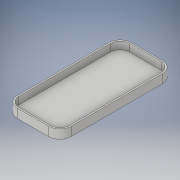
# Autodesk Inventor part: HandyHuelleMitText
Saved by Autodesk Inventor 2018 (Build 220112000, 112)
## iProperties
Created: 2017-06-18
Part Number: HandyHuelleMitText
Material: Generisch
Document SubType Name: Modeling
Designer: Ich
Density: 1 g/cm^3
Appearance: Vorgabe
Author: Ich
Autodesk Inventor part; units mm, degrees
ref_plane "YZ Plane" through (0, 0, 0) normal (1, 0, 0) x (0, 1, 0)
ref_plane "XZ Plane" through (0, 0, 0) normal (0, 1, 0) x (-1, 0, 0)
ref_plane "XY Plane" through (0, 0, 0) normal (0, 0, 1) x (1, 0, 0)
sketch "Skizze1" plane through (0, 0, 0) normal (0, 0, 1) x (1, 0, 0)
  line L0 (21, -76.5) -> (-21, -76.5)
  line L1 (-36, -61.5) -> (-36, 61.5)
  line L2 (-21, 76.5) -> (21, 76.5)
  line L3 (36, 61.5) -> (36, -61.5)
  line L4 (36, -76.5) -> (-36, 76.5) construction
  line L5 (-36, -76.5) -> (36, 76.5) construction
  arc A0 (-21, 76.5) -> (-36, 61.5) centre (-21, 61.5) ccw
  arc A1 (36, 61.5) -> (21, 76.5) centre (21, 61.5) ccw
  arc A2 (21, -76.5) -> (36, -61.5) centre (21, -61.5) ccw
  arc A3 (-36, -61.5) -> (-21, -76.5) centre (-21, -61.5) ccw
  point P0 (0, 0)
  dimension "d0" = 72
  dimension "d1" = 153
  dimension "d4" = 15
  dimension "d5" = 15
  constraints: 12 end point, 8 point on circle, 8 point on line, 8 tangent, 4 centre point, 2 equal radius, 2 midpoint, 2 parallel, 1 horizontal, 1 perpendicular
  measures "d0" distance between parallel lines of L3 L1
  measures "d1" distance between parallel lines of L0 L2
  measures "d4" radius of A0
  measures "d5" radius of A1
extrude "Extrusion1" add sketch "Skizze1" along normal blind 12
sketch "Skizze2" plane through (0, 0, 12) normal (0, 0, 1) x (1, 0, 0)
  line L0 (21, -74.5) -> (-21, -74.5)
  line L1 (-34, -61.5) -> (-34, 61.5)
  line L2 (-21, 74.5) -> (21, 74.5)
  line L3 (34, 61.5) -> (34, -61.5)
  line L4 (34, -74.5) -> (-34, 74.5) construction
  line L5 (-34, -74.5) -> (34, 74.5) construction
  arc A0 (34, 61.5) -> (21, 74.5) centre (21, 61.5) ccw
  arc A1 (-21, 74.5) -> (-34, 61.5) centre (-21, 61.5) ccw
  arc A2 (-34, -61.5) -> (-21, -74.5) centre (-21, -61.5) ccw
  arc A3 (21, -74.5) -> (34, -61.5) centre (21, -61.5) ccw
  point P0 (0, 0)
  dimension "d6" = 149
  dimension "d7" = 68
  dimension "d8" = 13
  constraints: 12 end point, 8 point on circle, 8 point on line, 8 tangent, 4 centre point, 3 equal radius, 2 midpoint, 2 parallel, 1 horizontal, 1 perpendicular
  measures "d6" distance between parallel lines of L0 L2
  measures "d7" distance between parallel lines of L1 L3
  measures "d8" radius of A0
extrude "Extrusion2" cut sketch "Skizze2" against normal blind 10
sketch "TextSkizze" plane through (0, 0, 0) normal (0, 0, -1) x (-1, 0, 0)
  line L0 (-11.4354, 0) -> (11.4354, 0) construction
  line L1 (11.4354, 0) -> (11.4354, -5.5416) construction
  line L2 (11.4354, -5.5416) -> (-11.4354, -5.5416) construction
  line L3 (-11.4354, -5.5416) -> (-11.4354, 0) construction
  line L4 (0, 88.5147) -> (0, -102.809) construction
  line L5 (-76.4782, 0) -> (138.3762, 0) construction
  line L6 (21, 76.5) -> (-21, 76.5) construction
  arc A0 (-21, 76.5) -> (-36, 61.5) centre (-21, 61.5) ccw construction
  line L7 (-36, 61.5) -> (-36, -61.5) construction
  arc A1 (-36, -61.5) -> (-21, -76.5) centre (-21, -61.5) ccw construction
  line L8 (-21, -76.5) -> (21, -76.5) construction
  arc A2 (21, -76.5) -> (36, -61.5) centre (21, -61.5) ccw construction
  line L9 (36, -61.5) -> (36, 61.5) construction
  arc A3 (36, 61.5) -> (21, 76.5) centre (21, 61.5) ccw construction
  line L10 (-10.2641, -3.5) -> (-10.2641, -0.4141)
  line L11 (-10.2641, -0.4141) -> (-11.4383, -0.4141)
  line L12 (-11.4383, -0.4141) -> (-11.4383, 0)
  line L13 (-11.4383, 0) -> (-8.6247, 0)
  line L14 (-8.6247, 0) -> (-8.6247, -0.4141)
  line L15 (-8.6247, -0.4141) -> (-9.7989, -0.4141)
  line L16 (-9.7989, -0.4141) -> (-9.7989, -3.5)
  line L17 (-9.7989, -3.5) -> (-10.2641, -3.5)
  spline S0 degree 2 poles (-7.164, -3.5596) (-7.7936, -3.5596) (-8.4857, -2.8533) (-8.4857, -2.201) knots 0 0 0 1 2 2 2
  spline S1 degree 2 poles (-8.4857, -2.201) (-8.4857, -1.56) (-7.8135, -0.7998) (-7.2717, -0.7998) knots 0 0 0 1 2 2 2
  spline S2 degree 2 poles (-7.2717, -0.7998) (-7.0278, -0.7998) (-6.6506, -0.9417) (-6.5116, -1.092) knots 0 0 0 1 2 2 2
  spline S3 degree 2 poles (-6.5116, -1.092) (-6.3698, -1.2423) (-6.2195, -1.6763) (-6.2195, -1.9911) knots 0 0 0 1 2 2 2
  line L18 (-6.2195, -1.9911) -> (-6.2195, -2.2322)
  line L19 (-6.2195, -2.2322) -> (-8.0376, -2.2322)
  spline S4 degree 2 poles (-8.0376, -2.2322) (-8.0376, -2.6888) (-7.5781, -3.1738) (-7.1696, -3.1738) knots 0 0 0 1 2 2 2
  spline S5 degree 2 poles (-7.1696, -3.1738) (-7.025, -3.1738) (-6.7442, -3.1086) (-6.6307, -3.0575) knots 0 0 0 1 2 2 2
  spline S6 degree 2 poles (-6.6307, -3.0575) (-6.5116, -3.0008) (-6.3471, -2.9015) (-6.2932, -2.8562) knots 0 0 0 1 2 2 2
  line L20 (-6.2932, -2.8562) -> (-6.2677, -2.8562)
  line L21 (-6.2677, -2.8562) -> (-6.2677, -3.3383)
  spline S7 degree 2 poles (-6.2677, -3.3383) (-6.3443, -3.3695) (-6.5769, -3.4603) (-6.6676, -3.4858) knots 0 0 0 1 2 2 2
  spline S8 degree 2 poles (-6.6676, -3.4858) (-6.7953, -3.5227) (-7.0051, -3.5596) (-7.164, -3.5596) knots 0 0 0 1 2 2 2
  spline S9 degree 2 poles (-6.6506, -1.8947) (-6.6563, -1.716) (-6.73, -1.455) (-6.8009, -1.3671) knots 0 0 0 1 2 2 2
  spline S10 degree 2 poles (-6.8009, -1.3671) (-6.8775, -1.2678) (-7.1186, -1.1629) (-7.2973, -1.1629) knots 0 0 0 1 2 2 2
  spline S11 degree 2 poles (-7.2973, -1.1629) (-7.4731, -1.1629) (-7.7199, -1.2678) (-7.822, -1.3699) knots 0 0 0 1 2 2 2
  spline S12 degree 2 poles (-7.822, -1.3699) (-7.9213, -1.4749) (-8.0234, -1.7273) (-8.0376, -1.8947) knots 0 0 0 1 2 2 2
  line L22 (-8.0376, -1.8947) -> (-6.6506, -1.8947)
  spline S13 degree 2 poles (-5.0623, -3.5624) (-5.326, -3.5624) (-5.7827, -3.4206) (-5.933, -3.3412) knots 0 0 0 1 2 2 2
  line L23 (-5.933, -3.3412) -> (-5.933, -2.8448)
  line L24 (-5.933, -2.8448) -> (-5.9103, -2.8448)
  spline S14 degree 2 poles (-5.9103, -2.8448) (-5.8536, -2.8902) (-5.7004, -2.998) (-5.5728, -3.0575) knots 0 0 0 1 2 2 2
  spline S15 degree 2 poles (-5.5728, -3.0575) (-5.4622, -3.1114) (-5.1899, -3.1908) (-5.0453, -3.1908) knots 0 0 0 1 2 2 2
  spline S16 degree 2 poles (-5.0453, -3.1908) (-4.9403, -3.1908) (-4.6992, -3.1426) (-4.6425, -3.1029) knots 0 0 0 1 2 2 2
  spline S17 degree 2 poles (-4.6425, -3.1029) (-4.5602, -3.049) (-4.4865, -2.9271) (-4.4865, -2.8023) knots 0 0 0 1 2 2 2
  spline S18 degree 2 poles (-4.4865, -2.8023) (-4.4865, -2.6463) (-4.6567, -2.4846) (-4.8751, -2.4307) knots 0 0 0 1 2 2 2
  spline S19 degree 2 poles (-4.8751, -2.4307) (-4.9602, -2.4109) (-5.2324, -2.3541) (-5.3487, -2.3229) knots 0 0 0 1 2 2 2
  spline S20 degree 2 poles (-5.3487, -2.3229) (-5.6494, -2.235) (-5.9217, -1.872) (-5.9217, -1.6139) knots 0 0 0 1 2 2 2
  spline S21 degree 2 poles (-5.9217, -1.6139) (-5.9217, -1.2565) (-5.3856, -0.8112) (-4.9431, -0.8112) knots 0 0 0 1 2 2 2
  spline S22 degree 2 poles (-4.9431, -0.8112) (-4.7247, -0.8112) (-4.2823, -0.919) (-4.132, -1.0012) knots 0 0 0 1 2 2 2
  line L25 (-4.132, -1.0012) -> (-4.132, -1.4749)
  line L26 (-4.132, -1.4749) -> (-4.1547, -1.4749)
  spline S23 degree 2 poles (-4.1547, -1.4749) (-4.3248, -1.3387) (-4.7389, -1.1827) (-4.9517, -1.1827) knots 0 0 0 1 2 2 2
  spline S24 degree 2 poles (-4.9517, -1.1827) (-5.17, -1.1827) (-5.4707, -1.3671) (-5.4707, -1.5515) knots 0 0 0 1 2 2 2
  spline S25 degree 2 poles (-5.4707, -1.5515) (-5.4707, -1.7188) (-5.292, -1.8805) (-5.0935, -1.9315) knots 0 0 0 1 2 2 2
  spline S26 degree 2 poles (-5.0935, -1.9315) (-4.997, -1.9571) (-4.7531, -2.0081) (-4.6198, -2.0393) knots 0 0 0 1 2 2 2
  spline S27 degree 2 poles (-4.6198, -2.0393) (-4.3305, -2.113) (-4.0355, -2.4506) (-4.0355, -2.7427) knots 0 0 0 1 2 2 2
  spline S28 degree 2 poles (-4.0355, -2.7427) (-4.0355, -2.9129) (-4.1688, -3.2135) (-4.2993, -3.3241) knots 0 0 0 1 2 2 2
  spline S29 degree 2 poles (-4.2993, -3.3241) (-4.4383, -3.4404) (-4.7928, -3.5624) (-5.0623, -3.5624) knots 0 0 0 1 2 2 2
  spline S30 degree 2 poles (-2.8301, -3.5511) (-3.1903, -3.5511) (-3.5959, -3.1398) (-3.5959, -2.6945) knots 0 0 0 1 2 2 2
  line L27 (-3.5959, -2.6945) -> (-3.5959, -1.2395)
  line L28 (-3.5959, -1.2395) -> (-3.8937, -1.2395)
  line L29 (-3.8937, -1.2395) -> (-3.8937, -0.8736)
  line L30 (-3.8937, -0.8736) -> (-3.5959, -0.8736)
  line L31 (-3.5959, -0.8736) -> (-3.5959, -0.1191)
  line L32 (-3.5959, -0.1191) -> (-3.1534, -0.1191)
  line L33 (-3.1534, -0.1191) -> (-3.1534, -0.8736)
  line L34 (-3.1534, -0.8736) -> (-2.3394, -0.8736)
  line L35 (-2.3394, -0.8736) -> (-2.3394, -1.2395)
  line L36 (-2.3394, -1.2395) -> (-3.1534, -1.2395)
  line L37 (-3.1534, -1.2395) -> (-3.1534, -2.4903)
  spline S31 degree 2 poles (-3.1534, -2.4903) (-3.1534, -2.6888) (-3.1393, -2.9072) (-3.091, -3.0008) knots 0 0 0 1 2 2 2
  spline S32 degree 2 poles (-3.091, -3.0008) (-3.0513, -3.0831) (-2.8726, -3.1653) (-2.7195, -3.1653) knots 0 0 0 1 2 2 2
  spline S33 degree 2 poles (-2.7195, -3.1653) (-2.6117, -3.1653) (-2.4103, -3.1001) (-2.3649, -3.0802) knots 0 0 0 1 2 2 2
  line L38 (-2.3649, -3.0802) -> (-2.3394, -3.0802)
  line L39 (-2.3394, -3.0802) -> (-2.3394, -3.4773)
  spline S34 degree 2 poles (-2.3394, -3.4773) (-2.4642, -3.5113) (-2.7195, -3.5511) (-2.8301, -3.5511) knots 0 0 0 1 2 2 2
  line L40 (-1.1623, -3.5) -> (-1.1623, -0.4141)
  line L41 (-1.1623, -0.4141) -> (-2.3366, -0.4141)
  line L42 (-2.3366, -0.4141) -> (-2.3366, 0)
  line L43 (-2.3366, 0) -> (0.477, 0)
  line L44 (0.477, 0) -> (0.477, -0.4141)
  line L45 (0.477, -0.4141) -> (-0.6972, -0.4141)
  line L46 (-0.6972, -0.4141) -> (-0.6972, -3.5)
  line L47 (-0.6972, -3.5) -> (-1.1623, -3.5)
  spline S35 degree 2 poles (1.9377, -3.5596) (1.3081, -3.5596) (0.616, -2.8533) (0.616, -2.201) knots 0 0 0 1 2 2 2
  spline S36 degree 2 poles (0.616, -2.201) (0.616, -1.56) (1.2882, -0.7998) (1.83, -0.7998) knots 0 0 0 1 2 2 2
  spline S37 degree 2 poles (1.83, -0.7998) (2.0739, -0.7998) (2.4511, -0.9417) (2.5901, -1.092) knots 0 0 0 1 2 2 2
  spline S38 degree 2 poles (2.5901, -1.092) (2.7319, -1.2423) (2.8822, -1.6763) (2.8822, -1.9911) knots 0 0 0 1 2 2 2
  line L48 (2.8822, -1.9911) -> (2.8822, -2.2322)
  line L49 (2.8822, -2.2322) -> (1.0642, -2.2322)
  spline S39 degree 2 poles (1.0642, -2.2322) (1.0642, -2.6888) (1.5236, -3.1738) (1.9321, -3.1738) knots 0 0 0 1 2 2 2
  spline S40 degree 2 poles (1.9321, -3.1738) (2.0767, -3.1738) (2.3575, -3.1086) (2.471, -3.0575) knots 0 0 0 1 2 2 2
  spline S41 degree 2 poles (2.471, -3.0575) (2.5901, -3.0008) (2.7546, -2.9015) (2.8085, -2.8562) knots 0 0 0 1 2 2 2
  line L50 (2.8085, -2.8562) -> (2.834, -2.8562)
  line L51 (2.834, -2.8562) -> (2.834, -3.3383)
  spline S42 degree 2 poles (2.834, -3.3383) (2.7574, -3.3695) (2.5248, -3.4603) (2.4341, -3.4858) knots 0 0 0 1 2 2 2
  spline S43 degree 2 poles (2.4341, -3.4858) (2.3065, -3.5227) (2.0966, -3.5596) (1.9377, -3.5596) knots 0 0 0 1 2 2 2
  spline S44 degree 2 poles (2.4511, -1.8947) (2.4454, -1.716) (2.3717, -1.455) (2.3008, -1.3671) knots 0 0 0 1 2 2 2
  spline S45 degree 2 poles (2.3008, -1.3671) (2.2242, -1.2678) (1.9831, -1.1629) (1.8044, -1.1629) knots 0 0 0 1 2 2 2
  spline S46 degree 2 poles (1.8044, -1.1629) (1.6286, -1.1629) (1.3818, -1.2678) (1.2797, -1.3699) knots 0 0 0 1 2 2 2
  spline S47 degree 2 poles (1.2797, -1.3699) (1.1804, -1.4749) (1.0783, -1.7273) (1.0642, -1.8947) knots 0 0 0 1 2 2 2
  line L52 (1.0642, -1.8947) -> (2.4511, -1.8947)
  line L53 (5.3697, -3.5) -> (4.8279, -3.5)
  line L54 (4.8279, -3.5) -> (4.1898, -2.513)
  line L55 (4.1898, -2.513) -> (3.5346, -3.5)
  line L56 (3.5346, -3.5) -> (3.0325, -3.5)
  line L57 (3.0325, -3.5) -> (3.943, -2.1981)
  line L58 (3.943, -2.1981) -> (3.0411, -0.8736)
  line L59 (3.0411, -0.8736) -> (3.5828, -0.8736)
  line L60 (3.5828, -0.8736) -> (4.2181, -1.8521)
  line L61 (4.2181, -1.8521) -> (4.8676, -0.8736)
  line L62 (4.8676, -0.8736) -> (5.3697, -0.8736)
  line L63 (5.3697, -0.8736) -> (4.4649, -2.1698)
  line L64 (4.4649, -2.1698) -> (5.3697, -3.5)
  spline S48 degree 2 poles (6.507, -3.5511) (6.1468, -3.5511) (5.7412, -3.1398) (5.7412, -2.6945) knots 0 0 0 1 2 2 2
  line L65 (5.7412, -2.6945) -> (5.7412, -1.2395)
  line L66 (5.7412, -1.2395) -> (5.4434, -1.2395)
  line L67 (5.4434, -1.2395) -> (5.4434, -0.8736)
  line L68 (5.4434, -0.8736) -> (5.7412, -0.8736)
  line L69 (5.7412, -0.8736) -> (5.7412, -0.1191)
  line L70 (5.7412, -0.1191) -> (6.1837, -0.1191)
  line L71 (6.1837, -0.1191) -> (6.1837, -0.8736)
  line L72 (6.1837, -0.8736) -> (6.9977, -0.8736)
  line L73 (6.9977, -0.8736) -> (6.9977, -1.2395)
  line L74 (6.9977, -1.2395) -> (6.1837, -1.2395)
  line L75 (6.1837, -1.2395) -> (6.1837, -2.4903)
  spline S49 degree 2 poles (6.1837, -2.4903) (6.1837, -2.6888) (6.1979, -2.9072) (6.2461, -3.0008) knots 0 0 0 1 2 2 2
  spline S50 degree 2 poles (6.2461, -3.0008) (6.2858, -3.0831) (6.4645, -3.1653) (6.6176, -3.1653) knots 0 0 0 1 2 2 2
  spline S51 degree 2 poles (6.6176, -3.1653) (6.7254, -3.1653) (6.9268, -3.1001) (6.9722, -3.0802) knots 0 0 0 1 2 2 2
  line L76 (6.9722, -3.0802) -> (6.9977, -3.0802)
  line L77 (6.9977, -3.0802) -> (6.9977, -3.4773)
  spline S52 degree 2 poles (6.9977, -3.4773) (6.8729, -3.5113) (6.6176, -3.5511) (6.507, -3.5511) knots 0 0 0 1 2 2 2
  point P0 (0, 0)
  dimension "d11" = 76.5
  constraints: 4 end point, 1 collinear, 1 horizontal, 1 symmetric about line, 1 vertical, 2 other
  measures "d11" distance between parallel lines of L5 L6
emboss "Prägen1" sketch "TextSkizze" operation add depth 1 direction (0, 0, 1)
equation "\"d0\" = Breite"
equation "\"d1\" = Höhe"
equation "\"d2\" = Tiefe"
equation "\"d6\" = Höhe - 2 * Wandstärke"
equation "\"d7\" = Breite - 2 * Wandstärke"
equation "\"d9\" = Tiefe - Wandstärke"
equation "\"d11\" = 0.5 * Höhe"
equation "\"Wandstärke\" = 2"
equation "\"Breite\" = 72"
equation "\"Höhe\" = 153"
equation "\"Tiefe\" = 12"
